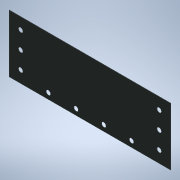
# Autodesk Inventor part: New side
Saved by Autodesk Inventor 2020 (Build 240168000, 168)
## iProperties
Created: 2022-07-17
Part Number: New side
Material: Generic
Document SubType Name: Sheet Metal
Designer: karimi2
Density: 1 g/cm^3
Sheet Metal Rule: Default_mm
Appearance: Gunmetal - Polished
Author: karimi2
Autodesk Inventor part; units mm, degrees
ref_plane "YZ Plane" through (0, 0, 0) normal (1, 0, 0) x (0, 1, 0)
ref_plane "XZ Plane" through (0, 0, 0) normal (0, 1, 0) x (-1, 0, 0)
ref_plane "XY Plane" through (0, 0, 0) normal (0, 0, 1) x (1, 0, 0)
sketch "Sketch1" plane through (0, 0, 0) normal (0, 0, 1) x (1, 0, 0)
  line L0 (-140, 30) -> (-140, 130)
  line L1 (-140, 130) -> (0, 130)
  line L2 (0, 130) -> (0, 0) construction
  line L3 (140, 30) -> (140, 130)
  line L4 (140, 130) -> (0, 130)
  line L5 (-140, 30) -> (-100, 30)
  line L6 (100, 30) -> (140, 30)
  line L7 (-100, 130) -> (-100, 30)
  line L8 (100, 130) -> (100, 30)
  line L9 (-100, 30) -> (100, 30)
  point P0 (-100, 30)
  point P1 (100, 30)
  dimension "d0" = 140
  dimension "d57" = 40
  dimension "d58" = 40
  dimension "d88" = 100
  measures "d0" distance of L0.end L1.end
  measures "d57" distance between parallel lines of L7 L0
  measures "d58" distance between parallel lines of L3 L8
  measures "d88" distance of L0.start L0.end
extrude "Plate3" add sketch "Sketch1" along normal blind 0.5
sketch "Sketch7" plane through (0, 0, 0.5) normal (0, 0, 1) x (1, 0, 0)
  line L0 (-140, 130) -> (140, 130) projected
  line L1 (-140, 30) -> (-140, 130) projected
  line L2 (140, 130) -> (140, 30) projected
  point P0 (0, 0)
  point P1 (-120, 110)
  point P2 (-120, 80)
  point P3 (-120, 50)
  point P4 (120, 110)
  point P5 (120, 80)
  point P6 (120, 50)
  dimension "d98" = 20
  dimension "d99" = 50
  dimension "d100" = 80
  dimension "d101" = 20
  dimension "d102" = 20
  dimension "d103" = 50
  dimension "d104" = 80
  dimension "d105" = 20
  constraints: 4 vertical alignment
  measures "d98" distance from line of L0 point (-120, 110)
  measures "d99" distance from line of point (-120, 80) L0
  measures "d100" distance from line of point (-120, 50) L0
  measures "d101" distance from line of L1 point (-120, 110)
  measures "d102" distance from line of L0 point (120, 110)
  measures "d103" distance from line of point (120, 80) L0
  measures "d104" distance from line of point (120, 50) L0
  measures "d105" distance from line of L2 point (120, 110)
hole "Hole6" at (-120, 110, 0.5) at (-120, 80, 0.5) at (-120, 50, 0.5) at (120, 110, 0.5) at (120, 80, 0.5) at (120, 50, 0.5) direction (0, 0, -1) diameter 8 end through all
sketch "Sketch8" plane through (0, 0, 0.5) normal (0, 0, 1) x (1, 0, 0)
  line L0 (0, -26) -> (0, 156) projected
  line L1 (140, 30) -> (-140, 30) projected
  point P0 (0, 0)
  point P1 (-72, 40)
  point P2 (-24, 40)
  point P3 (24, 40)
  point P4 (72, 40)
  dimension "d117" = 24
  dimension "d118" = 48
  dimension "d119" = 48
  dimension "d120" = 48
  dimension "d121" = 10
  constraints: 3 horizontal alignment
  measures "d117" distance from line of L0 point (-24, 40)
  measures "d118" distance of point (24, 40) point (-24, 40)
  measures "d119" distance of point (-72, 40) point (-24, 40)
  measures "d120" distance of point (72, 40) point (24, 40)
  measures "d121" distance from line of L1 point (72, 40)
hole "Hole7" at (-72, 40, 0.5) at (-24, 40, 0.5) at (24, 40, 0.5) at (72, 40, 0.5) direction (0, 0, -1) diameter 8 end through all
equation "\"d96\" = Thickness"
equation "\"d111\" = Thickness"
equation "\"d90\" = Thickness"
equation "\"BendRadius\" = Thickness"
equation "\"BendReliefWidth\" = Thickness"
equation "\"BendReliefDepth\" = 0.5 * Thickness"
equation "\"CornerReliefSize\" = 4 * Thickness"
equation "\"MinimumRemnant\" = 2 * Thickness"
equation "\"TransitionRadius\" = BendRadius"
equation "\"JacobiRadiusSize\" = BendRadius"
equation "\"GapSize\" = Thickness"
equation "\"Thickness\" = 0.5"
body "Solid3"
